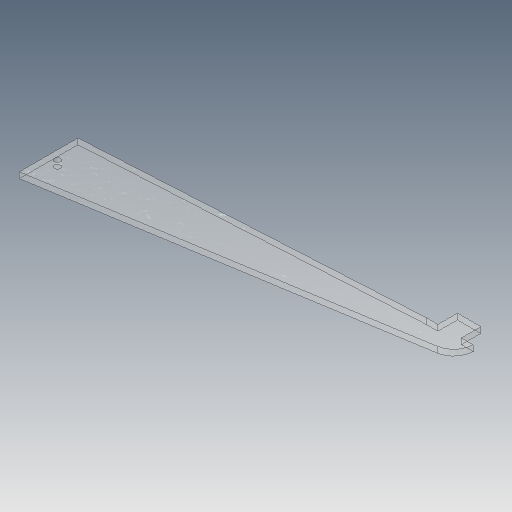
# Autodesk Inventor part: SqPipe92
Saved by Autodesk Inventor 2019.4 (Build 234330000, 330)
## iProperties
Created: 2019-06-12
Part Number: SqPipe92
Material: アクリル、クリア
Document SubType Name: Modeling
Designer: AzLIer
Density: 1.19 g/cm^3
Appearance: 透明 - クリア
Mass: 14.0257 g
Surface Area: 92.207 cm^2
Volume: 11.7863 cm^3
Author: AzLIer
Autodesk Inventor part; units mm, degrees
ref_plane "YZ Plane" through (0, 0, 0) normal (1, 0, 0) x (0, 1, 0)
ref_plane "XZ Plane" through (0, 0, 0) normal (0, 1, 0) x (-1, 0, 0)
ref_plane "XY Plane" through (0, 0, 0) normal (0, 0, 1) x (1, 0, 0)
sketch "スケッチ3" plane through (0, 0, 0) normal (0, 1, 0) x (-1, 0, 0)
  line L0 (0, -35.3598) -> (0, -5.3598)
  line L1 (-187, -44.8598) -> (-187, -54.8598) projected
  line L2 (-175, -44.8598) -> (-175, -54.8598) projected
  line L3 (0, -5.3598) -> (-184.5847, -34.9862)
  arc A0 (-184.5847, -34.9862) -> (-193, -44.8598) centre (-183, -44.8598) ccw
  line L4 (-187, -54.8598) -> (-175, -54.8598)
  line L5 (-187, -44.8598) -> (-193, -44.8598)
  line L6 (0, -35.3598) -> (-169, -44.8598)
  line L7 (-169, -44.8598) -> (-175, -44.8598)
  circle A1 centre (-4.5, -20.3598) radius 1.6 projected
  point P0 (0, -20.3598)
  dimension "d17" = 10
  dimension "d18" = 6
  dimension "d20" = 30
  dimension "d21" = 4.5
  constraints: 12 end point, 2 collinear, 2 horizontal, 2 point on circle, 1 centre point, 1 horizontal alignment, 1 line through centre, 1 midpoint, 1 tangent, 1 vertical
  measures "d17" radius of A0
  measures "d18" distance of L1.start L5.end
  measures "d20" distance of L0.start L0.end
  measures "d21" distance from line of A1.centre L0
extrude "押し出し2" add sketch "スケッチ3" along normal blind 3
